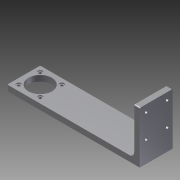
# Autodesk Inventor part: Einfach Nema
Saved by Autodesk Inventor 2011 (Build 150239000, 239)
## iProperties
Created: 2015-05-27
Part Number: Einfach Nema
Document SubType Name: Modeling
Designer: schmieder
Density: 1 g/cm^3
Author: schmieder
Autodesk Inventor part; units mm, degrees
ref_plane "YZ Plane" through (0, 0, 0) normal (1, 0, 0) x (0, 1, 0)
ref_plane "XZ Plane" through (0, 0, 0) normal (0, 1, 0) x (-1, 0, 0)
ref_plane "XY Plane" through (0, 0, 0) normal (0, 0, 1) x (1, 0, 0)
sketch "Skizze1" plane through (0, 0, 0) normal (0, 0, 1) x (1, 0, 0)
  line L0 (0, 0) -> (-35, 0)
  line L1 (-35, 0) -> (-35, 35)
  line L2 (-35, 35) -> (0, 35)
  line L3 (0, 35) -> (0, 0)
  dimension "d0" = 35
  dimension "d1" = 35
  constraints: 8 end point, 2 parallel, 1 horizontal, 1 perpendicular
  measures "d0" distance of L1.end L2.end
  measures "d1" distance of L0.end L1.end
extrude "NEMA11 Halter" add sketch "Skizze1" along normal blind 6
sketch "Skizze2" plane through (0, 0, 6) normal (0, 0, 1) x (1, 0, 0)
  circle A0 centre (-17.5, 17.5) radius 12.5
  dimension "d4" = 25
  constraints: 1 centre point
  measures "d4" diameter of A0
extrude "Motorloch" cut sketch "Skizze2" against normal up to surface (6 mm away)
sketch "Skizze3" plane through (0, 0, 6) normal (0, 0, 1) x (1, 0, 0)
  circle A0 centre (-29, 29) radius 1.4
  circle A1 centre (-17.5, 17.5) radius 12.5 projected
  line L0 (-35, 0) -> (-35, 35) projected
  line L1 (0, 0) -> (-35, 0) projected
  line L2 (0, 35) -> (0, 0) projected
  line L3 (-35, 35) -> (0, 35) projected
  circle A2 centre (-6, 29) radius 1.4
  circle A3 centre (-29, 6) radius 1.4
  circle A4 centre (-6, 6) radius 1.4
  dimension "d7" = 2.8
  dimension "d8" = 2.8
  dimension "d9" = 23
  dimension "d10" = 2.8
  dimension "d11" = 23
  dimension "d12" = 2.8
  dimension "d13" = 23
  dimension "d14" = 23
  constraints: 4 centre point
  measures "d7" diameter of A0
  measures "d8" diameter of A2
  measures "d9" distance of A2.centre A0.centre
  measures "d10" diameter of A3
  measures "d11" distance of A3.centre A0.centre
  measures "d12" diameter of A4
  measures "d13" distance of A4.centre A3.centre
  measures "d14" distance of A2.centre A4.centre
extrude "Motorschrauben" cut sketch "Skizze3" against normal up to surface (6 mm away) contours A0 | A2 | A3 | A4
sketch "Skizze22" plane through (0, 0, 6) normal (0, 0, 1) x (1, 0, 0)
  circle A0 centre (-6, 6) radius 1.4 projected
  circle A1 centre (-29, 29) radius 1.4 projected
  circle A2 centre (-6, 29) radius 1.4 projected
  circle A3 centre (-29, 6) radius 1.4 projected
  circle A4 centre (-29, 29) radius 2.5
  circle A5 centre (-6, 29) radius 2.5
  circle A6 centre (-6, 6) radius 2.5
  circle A7 centre (-29, 6) radius 2.5
  dimension "d78" = 5
  dimension "d79" = 5
  dimension "d80" = 5
  dimension "d81" = 5
  constraints: 4 centre point, 4 coincident
  measures "d78" diameter of A4
  measures "d79" diameter of A5
  measures "d80" diameter of A6
  measures "d81" diameter of A7
extrude "Extrusion16" cut sketch "Skizze22" against normal blind 1
sketch "Skizze23" plane through (0, 0, 6) normal (0, 0, 1) x (1, 0, 0)
  line L0 (0, 35) -> (100, 35)
  line L1 (100, 35) -> (100, 0)
  line L2 (100, 0) -> (0, 0)
  line L3 (0, 0) -> (0, 35)
  dimension "d84" = 100
  constraints: 8 end point, 2 parallel, 1 horizontal, 1 perpendicular
  measures "d84" distance of L1.end L2.end
extrude "Extrusion17" add sketch "Skizze23" against normal blind 6
sketch "Skizze24" plane through (-35, 0, 0) normal (0, -1, 0) x (1, 0, 0)
  line L0 (135, 0) -> (141, 0)
  line L1 (141, 0) -> (141, 55)
  line L2 (141, 55) -> (135, 55)
  line L3 (135, 55) -> (135, 0)
  point P0 (35, 0)
  dimension "d87" = 6
  dimension "d88" = 55
  constraints: 8 end point, 2 parallel, 1 horizontal, 1 perpendicular
  measures "d87" distance of L2.end L1.end
  measures "d88" distance of L1.end L0.end
extrude "Extrusion18" add sketch "Skizze24" against normal up to surface (35 mm away)
fillet "Rundung8" radius 5 1 edges at (100, 17.5, 6)
fillet "Rundung9" radius 1 2 edges at (103, 0, 55) (103, 35, 55)
fillet "Rundung10" radius 1 2 edges at (-35, 0, 3) (-35, 35, 3)
sketch "Skizze25" plane through (100, 0, 11) normal (-1, 0, 0) x (0, 0, 1)
  circle A0 centre (36.6571, 29.1388) radius 1.5
  circle A1 centre (36.6571, 6.8732) radius 1.5
  circle A2 centre (11.524, 29.1388) radius 1.5
  circle A3 centre (11.524, 6.8732) radius 1.5
  point P0 (-11, 0)
  dimension "d94" = 3
  dimension "d95" = 3
  dimension "d96" = 3
  dimension "d97" = 3
  constraints: 4 centre point
  measures "d94" diameter of A0
  measures "d95" diameter of A1
  measures "d96" diameter of A2
  measures "d97" diameter of A3
extrude "Extrusion19" cut sketch "Skizze25" against normal up to surface (6 mm away)
